Autodesk Inventor part; units mm, degrees
(part 2 of 3)
  line L885 (25.1106, 23.169) -> (25.1155, 23.1808)
  line L886 (25.1155, 23.1808) -> (25.12, 23.1924)
  line L887 (25.12, 23.1924) -> (25.124, 23.2037)
  line L888 (25.124, 23.2037) -> (25.1305, 23.2253)
  line L889 (25.1305, 23.2253) -> (25.1354, 23.2453)
  line L890 (25.1354, 23.2453) -> (25.1389, 23.2633)
  line L891 (25.1389, 23.2633) -> (25.1413, 23.2789)
  line L892 (25.1413, 23.2789) -> (25.1427, 23.2917)
  line L893 (25.1427, 23.2917) -> (25.1435, 23.3013)
  line L894 (25.1435, 23.3013) -> (25.1438, 23.3095)
  line L895 (25.1438, 23.3095) -> (25.1438, 23.4153)
  line L896 (25.1438, 23.4153) -> (25.1421, 23.4381)
  line L897 (25.1421, 23.4381) -> (25.138, 23.4642)
  line L898 (25.138, 23.4642) -> (25.1302, 23.498)
  line L899 (25.1302, 23.498) -> (25.1171, 23.5381)
  line L900 (25.1171, 23.5381) -> (25.0978, 23.5828)
  line L901 (25.0978, 23.5828) -> (25.0707, 23.6306)
  line L902 (25.0707, 23.6306) -> (25.0539, 23.6551)
  line L903 (25.0539, 23.6551) -> (25.0347, 23.6799)
  line L904 (25.0347, 23.6799) -> (25.0129, 23.7047)
  line L905 (25.0129, 23.7047) -> (24.9884, 23.7293)
  line L906 (24.9884, 23.7293) -> (24.961, 23.7535)
  line L907 (24.961, 23.7535) -> (24.9306, 23.7771)
  line L908 (24.9306, 23.7771) -> (24.897, 23.7999)
  line L909 (24.897, 23.7999) -> (24.8601, 23.8218)
  line L910 (24.8601, 23.8218) -> (24.8196, 23.8425)
  line L911 (24.8196, 23.8425) -> (24.7754, 23.8618)
  line L912 (24.7754, 23.8618) -> (24.7275, 23.8796)
  line L913 (24.7275, 23.8796) -> (24.6755, 23.8957)
  line L914 (24.6755, 23.8957) -> (24.6193, 23.9098)
  line L915 (24.6193, 23.9098) -> (24.5589, 23.9218)
  line L916 (24.5589, 23.9218) -> (24.4939, 23.9314)
  line L917 (24.4939, 23.9314) -> (24.4244, 23.9385)
  line L918 (24.4244, 23.9385) -> (24.35, 23.943)
  line L919 (24.35, 23.943) -> (24.2707, 23.9445)
  line L920 (24.2707, 23.9445) -> (21.0957, 23.9445)
  line L921 (21.0957, 23.9445) -> (21.0324, 23.9439)
  line L922 (21.0324, 23.9439) -> (20.9716, 23.9419)
  line L923 (20.9716, 23.9419) -> (20.9132, 23.9386)
  line L924 (20.9132, 23.9386) -> (20.8571, 23.9337)
  line L925 (20.8571, 23.9337) -> (20.8034, 23.9274)
  line L926 (20.8034, 23.9274) -> (20.752, 23.9194)
  line L927 (20.752, 23.9194) -> (20.7028, 23.9097)
  line L928 (20.7028, 23.9097) -> (20.6558, 23.8982)
  line L929 (20.6558, 23.8982) -> (20.611, 23.8848)
  line L930 (20.611, 23.8848) -> (20.5683, 23.8696)
  line L931 (20.5683, 23.8696) -> (20.5277, 23.8523)
  line L932 (20.5277, 23.8523) -> (20.4892, 23.8329)
  line L933 (20.4892, 23.8329) -> (20.4527, 23.8113)
  line L934 (20.4527, 23.8113) -> (20.4181, 23.7875)
  line L935 (20.4181, 23.7875) -> (20.3855, 23.7614)
  line L936 (20.3855, 23.7614) -> (20.3548, 23.7328)
  line L937 (20.3548, 23.7328) -> (20.3427, 23.7204)
  line L938 (20.3427, 23.7204) -> (20.3313, 23.7078)
  line L939 (20.3313, 23.7078) -> (20.3204, 23.6951)
  line L940 (20.3204, 23.6951) -> (20.31, 23.6823)
  line L941 (20.31, 23.6823) -> (20.3003, 23.6696)
  line L942 (20.3003, 23.6696) -> (20.2911, 23.6568)
  line L943 (20.2911, 23.6568) -> (20.2824, 23.6442)
  line L944 (20.2824, 23.6442) -> (20.2742, 23.6315)
  line L945 (20.2742, 23.6315) -> (20.2666, 23.619)
  line L946 (20.2666, 23.619) -> (20.2594, 23.6067)
  line L947 (20.2594, 23.6067) -> (20.2465, 23.5826)
  line L948 (20.2465, 23.5826) -> (20.2353, 23.5595)
  line L949 (20.2353, 23.5595) -> (20.2259, 23.5377)
  line L950 (20.2259, 23.5377) -> (20.2179, 23.5174)
  line L951 (20.2179, 23.5174) -> (20.2114, 23.499)
  line L952 (20.2114, 23.499) -> (20.2063, 23.4826)
  line L953 (20.2063, 23.4826) -> (20.2023, 23.4687)
  line L954 (20.2023, 23.4687) -> (20.1975, 23.4489)
  line L955 (20.1975, 23.4489) -> (20.1961, 23.4418)
  line L956 (20.1961, 23.4418) -> (20.1961, 22.8068)
  line L957 (19.7728, 22.8068) -> (19.7728, 23.4418)
  line L958 (19.7728, 23.4418) -> (19.7733, 23.4647)
  line L959 (19.7733, 23.4647) -> (19.7769, 23.5108)
  line L960 (19.7769, 23.5108) -> (19.7808, 23.5414)
  line L961 (19.7808, 23.5414) -> (19.7867, 23.5762)
  line L962 (19.7867, 23.5762) -> (19.7949, 23.6148)
  line L963 (19.7949, 23.6148) -> (19.8058, 23.6568)
  line L964 (19.8058, 23.6568) -> (19.8198, 23.7015)
  line L965 (19.8198, 23.7015) -> (19.8373, 23.7485)
  line L966 (19.8373, 23.7485) -> (19.8587, 23.7973)
  line L967 (19.8587, 23.7973) -> (19.8844, 23.8473)
  line L968 (19.8844, 23.8473) -> (19.9147, 23.8982)
  line L969 (19.9147, 23.8982) -> (19.95, 23.9493)
  line L970 (19.95, 23.9493) -> (19.9697, 23.9748)
  line L971 (19.9697, 23.9748) -> (19.9908, 24.0002)
  line L972 (19.9908, 24.0002) -> (20.0133, 24.0254)
  line L973 (20.0133, 24.0254) -> (20.0373, 24.0503)
  line L974 (20.0373, 24.0503) -> (20.0832, 24.0937)
  line L975 (20.0832, 24.0937) -> (20.1316, 24.1346)
  line L976 (20.1316, 24.1346) -> (20.1826, 24.1729)
  line L977 (20.1826, 24.1729) -> (20.2362, 24.2087)
  line L978 (20.2362, 24.2087) -> (20.2924, 24.2418)
  line L979 (20.2924, 24.2418) -> (20.3513, 24.2722)
  line L980 (20.3513, 24.2722) -> (20.4129, 24.2999)
  line L981 (20.4129, 24.2999) -> (20.4772, 24.3248)
  line L982 (20.4772, 24.3248) -> (20.5443, 24.347)
  line L983 (20.5443, 24.347) -> (20.6143, 24.3663)
  line L984 (20.6143, 24.3663) -> (20.6871, 24.3828)
  line L985 (20.6871, 24.3828) -> (20.7629, 24.3964)
  line L986 (20.7629, 24.3964) -> (20.8416, 24.407)
  line L987 (20.8416, 24.407) -> (20.9232, 24.4146)
  line L988 (20.9232, 24.4146) -> (21.0079, 24.4192)
  line L989 (21.0079, 24.4192) -> (21.0957, 24.4207)
  line L990 (21.0957, 24.4207) -> (24.2707, 24.4207)
  line L991 (24.2707, 24.4207) -> (24.3587, 24.4192)
  line L992 (28.4246, 20.8753) -> (27.9748, 20.8753)
  line L993 (27.9748, 20.8753) -> (27.9748, 23.6799)
  line L994 (27.9748, 23.6799) -> (26.7842, 22.3041)
  line L995 (26.7842, 22.3041) -> (26.2021, 22.3041)
  line L996 (26.2021, 22.3041) -> (28.0278, 24.3943)
  line L997 (28.0278, 24.3943) -> (28.4246, 24.3943)
  line L998 (28.4246, 24.3943) -> (28.4246, 20.8753)
  line L999 (36.3621, 21.4045) -> (40.86, 24.3149)
  line L1000 (40.86, 24.3149) -> (41.0982, 23.9445)
  line L1001 (41.0982, 23.9445) -> (38.9286, 22.5157)
  line L1002 (38.9286, 22.5157) -> (41.0982, 21.1135)
  line L1003 (41.0982, 21.1135) -> (40.86, 20.743)
  line L1004 (40.86, 20.743) -> (38.5317, 22.2512)
  line L1005 (38.5317, 22.2512) -> (35.9123, 20.5843)
  line L1006 (35.9123, 20.5843) -> (35.9123, 24.3943)
  line L1007 (35.9123, 24.3943) -> (36.3621, 24.3943)
  line L1008 (36.3621, 24.3943) -> (36.3621, 21.4045)
  line L1009 (42.2056, 21.9858) -> (42.2536, 21.9836)
  line L1010 (42.2536, 21.9836) -> (42.3006, 21.9799)
  line L1011 (42.3006, 21.9799) -> (42.3465, 21.9748)
  line L1012 (42.3465, 21.9748) -> (42.3915, 21.9684)
  line L1013 (42.3915, 21.9684) -> (42.4355, 21.9608)
  line L1014 (42.4355, 21.9608) -> (42.4786, 21.9519)
  line L1015 (42.4786, 21.9519) -> (42.5207, 21.9419)
  line L1016 (42.5207, 21.9419) -> (42.6024, 21.9188)
  line L1017 (42.6024, 21.9188) -> (42.6807, 21.8917)
  line L1018 (42.6807, 21.8917) -> (42.7558, 21.8612)
  line L1019 (42.7558, 21.8612) -> (42.8279, 21.8278)
  line L1020 (42.8279, 21.8278) -> (42.8972, 21.7919)
  line L1021 (42.8972, 21.7919) -> (42.9639, 21.754)
  line L1022 (42.9639, 21.754) -> (43.0283, 21.7146)
  line L1023 (43.0283, 21.7146) -> (43.0904, 21.674)
  line L1024 (43.0904, 21.674) -> (43.2088, 21.5916)
  line L1025 (43.2088, 21.5916) -> (43.3207, 21.5103)
  line L1026 (43.3207, 21.5103) -> (43.4077, 21.4435)
  line L1027 (43.4077, 21.4435) -> (43.491, 21.3826)
  line L1028 (43.491, 21.3826) -> (43.5316, 21.3546)
  line L1029 (43.5316, 21.3546) -> (43.5718, 21.3285)
  line L1030 (43.5718, 21.3285) -> (43.6117, 21.3043)
  line L1031 (43.6117, 21.3043) -> (43.6514, 21.2821)
  line L1032 (43.6514, 21.2821) -> (43.6911, 21.2621)
  line L1033 (43.6911, 21.2621) -> (43.731, 21.2444)
  line L1034 (43.731, 21.2444) -> (43.7712, 21.2292)
  line L1035 (43.7712, 21.2292) -> (43.8118, 21.2164)
  line L1036 (43.8118, 21.2164) -> (43.8531, 21.2063)
  line L1037 (43.8531, 21.2063) -> (43.8951, 21.1989)
  line L1038 (43.8951, 21.1989) -> (43.9381, 21.1944)
  line L1039 (43.9381, 21.1944) -> (43.9821, 21.1928)
  line L1040 (43.9821, 21.1928) -> (44.0262, 21.1944)
  line L1041 (44.0262, 21.1944) -> (44.0692, 21.1989)
  line L1042 (44.0692, 21.1989) -> (44.1112, 21.2063)
  line L1043 (44.1112, 21.2063) -> (44.1525, 21.2164)
  line L1044 (44.1525, 21.2164) -> (44.1931, 21.2292)
  line L1045 (44.1931, 21.2292) -> (44.2333, 21.2444)
  line L1046 (44.2333, 21.2444) -> (44.2731, 21.2621)
  line L1047 (44.2731, 21.2621) -> (44.3129, 21.2821)
  line L1048 (44.3129, 21.2821) -> (44.3526, 21.3043)
  line L1049 (44.3526, 21.3043) -> (44.3924, 21.3285)
  line L1050 (44.3924, 21.3285) -> (44.4326, 21.3546)
  line L1051 (44.4326, 21.3546) -> (44.4733, 21.3826)
  line L1052 (44.4733, 21.3826) -> (44.5566, 21.4435)
  line L1053 (44.5566, 21.4435) -> (44.6436, 21.5103)
  line L1054 (44.6436, 21.5103) -> (44.7554, 21.5916)
  line L1055 (44.7554, 21.5916) -> (44.873, 21.674)
  line L1056 (44.873, 21.674) -> (44.9344, 21.7146)
  line L1057 (44.9344, 21.7146) -> (44.9975, 21.754)
  line L1058 (44.9975, 21.754) -> (45.0626, 21.7919)
  line L1059 (45.0626, 21.7919) -> (45.1298, 21.8278)
  line L1060 (45.1298, 21.8278) -> (45.1991, 21.8612)
  line L1061 (45.1991, 21.8612) -> (45.2707, 21.8917)
  line L1062 (45.2707, 21.8917) -> (45.3447, 21.9188)
  line L1063 (45.3447, 21.9188) -> (45.4212, 21.9419)
  line L1064 (45.4212, 21.9419) -> (45.5004, 21.9608)
  line L1065 (45.5004, 21.9608) -> (45.5823, 21.9748)
  line L1066 (45.5823, 21.9748) -> (45.6671, 21.9836)
  line L1067 (45.6671, 21.9836) -> (45.7548, 21.9866)
  line L1068 (45.7548, 21.9866) -> (46.2575, 21.9866)
  line L1069 (46.2575, 21.9866) -> (46.2575, 21.5368)
  line L1070 (46.2575, 21.5368) -> (45.7548, 21.5368)
  line L1071 (45.7548, 21.5368) -> (45.7228, 21.5362)
  line L1072 (45.7228, 21.5362) -> (45.6913, 21.5344)
  line L1073 (45.6913, 21.5344) -> (45.6601, 21.5314)
  line L1074 (45.6601, 21.5314) -> (45.6294, 21.5273)
  line L1075 (45.6294, 21.5273) -> (45.5991, 21.5222)
  line L1076 (45.5991, 21.5222) -> (45.5692, 21.516)
  line L1077 (45.5692, 21.516) -> (45.5105, 21.5008)
  line L1078 (45.5105, 21.5008) -> (45.4532, 21.482)
  line L1079 (45.4532, 21.482) -> (45.3972, 21.46)
  line L1080 (45.3972, 21.46) -> (45.3423, 21.4352)
  line L1081 (45.3423, 21.4352) -> (45.2885, 21.4078)
  line L1082 (45.2885, 21.4078) -> (45.2356, 21.3782)
  line L1083 (45.2356, 21.3782) -> (45.1836, 21.3469)
  line L1084 (45.1836, 21.3469) -> (45.1322, 21.314)
  line L1085 (45.1322, 21.314) -> (45.0814, 21.2801)
  line L1086 (45.0814, 21.2801) -> (44.8817, 21.1399)
  line L1087 (44.8817, 21.1399) -> (44.7822, 21.0621)
  line L1088 (44.7822, 21.0621) -> (44.732, 21.0247)
  line L1089 (44.732, 21.0247) -> (44.6812, 20.9886)
  line L1090 (44.6812, 20.9886) -> (44.6296, 20.9541)
  line L1091 (44.6296, 20.9541) -> (44.5771, 20.9213)
  line L1092 (44.5771, 20.9213) -> (44.5234, 20.8906)
  line L1093 (44.5234, 20.8906) -> (44.4683, 20.8621)
  line L1094 (44.4683, 20.8621) -> (44.4117, 20.8361)
  line L1095 (44.4117, 20.8361) -> (44.3533, 20.8128)
  line L1096 (44.3533, 20.8128) -> (44.293, 20.7924)
  line L1097 (44.293, 20.7924) -> (44.2306, 20.7753)
  line L1098 (44.2306, 20.7753) -> (44.1658, 20.7615)
  line L1099 (44.1658, 20.7615) -> (44.0986, 20.7514)
  line L1100 (44.0986, 20.7514) -> (44.0286, 20.7452)
  line L1101 (44.0286, 20.7452) -> (43.9557, 20.743)
  line L1102 (43.9557, 20.743) -> (43.9188, 20.7436)
  line L1103 (43.9188, 20.7436) -> (43.8828, 20.7455)
  line L1104 (43.8828, 20.7455) -> (43.8474, 20.7484)
  line L1105 (43.8474, 20.7484) -> (43.8128, 20.7525)
  line L1106 (43.8128, 20.7525) -> (43.7788, 20.7576)
  line L1107 (43.7788, 20.7576) -> (43.7455, 20.7638)
  line L1108 (43.7455, 20.7638) -> (43.6808, 20.779)
  line L1109 (43.6808, 20.779) -> (43.6183, 20.7978)
  line L1110 (43.6183, 20.7978) -> (43.558, 20.8198)
  line L1111 (43.558, 20.8198) -> (43.4997, 20.8446)
  line L1112 (43.4997, 20.8446) -> (43.443, 20.872)
  line L1113 (43.443, 20.872) -> (43.388, 20.9016)
  line L1114 (43.388, 20.9016) -> (43.3343, 20.9329)
  line L1115 (43.3343, 20.9329) -> (43.2817, 20.9658)
  line L1116 (43.2817, 20.9658) -> (43.2301, 20.9998)
  line L1117 (43.2301, 20.9998) -> (43.1291, 21.0697)
  line L1118 (43.1291, 21.0697) -> (43.0296, 21.1399)
  line L1119 (43.0296, 21.1399) -> (42.9313, 21.2177)
  line L1120 (42.9313, 21.2177) -> (42.8337, 21.2912)
  line L1121 (42.8337, 21.2912) -> (42.7845, 21.3257)
  line L1122 (42.7845, 21.3257) -> (42.7348, 21.3585)
  line L1123 (42.7348, 21.3585) -> (42.6843, 21.3892)
  line L1124 (42.6843, 21.3892) -> (42.6328, 21.4177)
  line L1125 (42.6328, 21.4177) -> (42.58, 21.4437)
  line L1126 (42.58, 21.4437) -> (42.5258, 21.467)
  line L1127 (42.5258, 21.467) -> (42.4699, 21.4874)
  line L1128 (42.4699, 21.4874) -> (42.412, 21.5045)
  line L1129 (42.412, 21.5045) -> (42.352, 21.5183)
  line L1130 (42.352, 21.5183) -> (42.2895, 21.5284)
  line L1131 (42.2895, 21.5284) -> (42.2244, 21.5347)
  line L1132 (42.2244, 21.5347) -> (42.1565, 21.5368)
  line L1133 (42.1565, 21.5368) -> (41.6538, 21.5368)
  line L1134 (41.6538, 21.5368) -> (41.6538, 21.9866)
  line L1135 (41.6538, 21.9866) -> (42.1565, 21.9866)
  line L1136 (42.1565, 21.9866) -> (42.2056, 21.9858)
  line L1137 (35.2244, 23.9974) -> (29.9592, 23.9974)
  line L1138 (29.9592, 23.9974) -> (29.9942, 23.8886)
  line L1139 (29.9942, 23.8886) -> (30.0411, 23.7622)
  line L1140 (30.0411, 23.7622) -> (30.1015, 23.6202)
  line L1141 (30.1015, 23.6202) -> (30.1375, 23.5441)
  line L1142 (30.1375, 23.5441) -> (30.1775, 23.4649)
  line L1143 (30.1775, 23.4649) -> (30.2219, 23.383)
  line L1144 (30.2219, 23.383) -> (30.2708, 23.2985)
  line L1145 (30.2708, 23.2985) -> (30.3246, 23.2118)
  line L1146 (30.3246, 23.2118) -> (30.3834, 23.123)
  line L1147 (30.3834, 23.123) -> (30.4474, 23.0326)
  line L1148 (30.4474, 23.0326) -> (30.517, 22.9408)
  line L1149 (30.517, 22.9408) -> (30.5923, 22.8478)
  line L1150 (30.5923, 22.8478) -> (30.6736, 22.7539)
  line L1151 (30.6736, 22.7539) -> (30.7495, 22.6708)
  line L1152 (30.7495, 22.6708) -> (30.8286, 22.5902)
  line L1153 (30.8286, 22.5902) -> (30.9106, 22.512)
  line L1154 (30.9106, 22.512) -> (30.9956, 22.4364)
  line L1155 (30.9956, 22.4364) -> (31.0836, 22.3632)
  line L1156 (31.0836, 22.3632) -> (31.1745, 22.2925)
  line L1157 (31.1745, 22.2925) -> (31.2682, 22.2243)
  line L1158 (31.2682, 22.2243) -> (31.3648, 22.1586)
  line L1159 (31.3648, 22.1586) -> (31.4642, 22.0953)
  line L1160 (31.4642, 22.0953) -> (31.5663, 22.0345)
  line L1161 (31.5663, 22.0345) -> (31.6711, 21.9762)
  line L1162 (31.6711, 21.9762) -> (31.7786, 21.9204)
  line L1163 (31.7786, 21.9204) -> (31.8888, 21.8671)
  line L1164 (31.8888, 21.8671) -> (32.0015, 21.8163)
  line L1165 (32.0015, 21.8163) -> (32.1168, 21.7679)
  line L1166 (32.1168, 21.7679) -> (32.2346, 21.722)
  line L1167 (32.2346, 21.722) -> (32.5485, 21.6092)
  line L1168 (32.5485, 21.6092) -> (32.8754, 21.5095)
  line L1169 (32.8754, 21.5095) -> (33.0439, 21.4647)
  line L1170 (33.0439, 21.4647) -> (33.216, 21.4234)
  line L1171 (33.216, 21.4234) -> (33.3915, 21.3857)
  line L1172 (33.3915, 21.3857) -> (33.5708, 21.3516)
  line L1173 (33.5708, 21.3516) -> (33.7537, 21.3212)
  line L1174 (33.7537, 21.3212) -> (33.9405, 21.2946)
  line L1175 (33.9405, 21.2946) -> (34.1311, 21.2719)
  line L1176 (34.1311, 21.2719) -> (34.3257, 21.2532)
  line L1177 (34.3257, 21.2532) -> (34.5243, 21.2385)
  line L1178 (34.5243, 21.2385) -> (34.727, 21.2279)
  line L1179 (34.727, 21.2279) -> (34.9339, 21.2214)
  line L1180 (34.9339, 21.2214) -> (35.145, 21.2193)
  line L1181 (35.145, 21.2193) -> (35.2509, 21.2193)
  line L1182 (35.2509, 21.2193) -> (35.2509, 20.7695)
  line L1183 (35.2509, 20.7695) -> (35.145, 20.7695)
  line L1184 (35.145, 20.7695) -> (34.9283, 20.7717)
  line L1185 (34.9283, 20.7717) -> (34.7147, 20.7781)
  line L1186 (34.7147, 20.7781) -> (34.5043, 20.7889)
  line L1187 (34.5043, 20.7889) -> (34.2971, 20.8038)
  line L1188 (34.2971, 20.8038) -> (34.0932, 20.8229)
  line L1189 (34.0932, 20.8229) -> (33.8926, 20.8462)
  line L1190 (33.8926, 20.8462) -> (33.6953, 20.8736)
  line L1191 (33.6953, 20.8736) -> (33.5013, 20.9051)
  line L1192 (33.5013, 20.9051) -> (33.3108, 20.9406)
  line L1193 (33.3108, 20.9406) -> (33.1237, 20.9801)
  line L1194 (33.1237, 20.9801) -> (32.9401, 21.0235)
  line L1195 (32.9401, 21.0235) -> (32.7601, 21.0709)
  line L1196 (32.7601, 21.0709) -> (32.5836, 21.1221)
  line L1197 (32.5836, 21.1221) -> (32.4107, 21.1772)
  line L1198 (32.4107, 21.1772) -> (32.2414, 21.236)
  line L1199 (32.2414, 21.236) -> (32.0759, 21.2987)
  line L1200 (32.0759, 21.2987) -> (31.9438, 21.3542)
  line L1201 (31.9438, 21.3542) -> (31.8153, 21.4116)
  line L1202 (31.8153, 21.4116) -> (31.6904, 21.4711)
  line L1203 (31.6904, 21.4711) -> (31.569, 21.5327)
  line L1204 (31.569, 21.5327) -> (31.451, 21.5964)
  line L1205 (31.451, 21.5964) -> (31.3364, 21.6624)
  line L1206 (31.3364, 21.6624) -> (31.225, 21.7307)
  line L1207 (31.225, 21.7307) -> (31.1168, 21.8014)
  line L1208 (31.1168, 21.8014) -> (31.0116, 21.8746)
  line L1209 (31.0116, 21.8746) -> (30.9095, 21.9503)
  line L1210 (30.9095, 21.9503) -> (30.8104, 22.0287)
  line L1211 (30.8104, 22.0287) -> (30.7141, 22.1098)
  line L1212 (30.7141, 22.1098) -> (30.6206, 22.1937)
  line L1213 (30.6206, 22.1937) -> (30.5298, 22.2804)
  line L1214 (30.5298, 22.2804) -> (30.4417, 22.3701)
  line L1215 (30.4417, 22.3701) -> (30.3561, 22.4628)
  line L1216 (30.3561, 22.4628) -> (30.2861, 22.5422)
  line L1217 (30.2861, 22.5422) -> (30.2198, 22.6214)
  line L1218 (30.2198, 22.6214) -> (30.1573, 22.7003)
  line L1219 (30.1573, 22.7003) -> (30.0983, 22.7787)
  line L1220 (30.0983, 22.7787) -> (30.0427, 22.8566)
  line L1221 (30.0427, 22.8566) -> (29.9906, 22.9337)
  line L1222 (29.9906, 22.9337) -> (29.9417, 23.0099)
  line L1223 (29.9417, 23.0099) -> (29.896, 23.085)
  line L1224 (29.896, 23.085) -> (29.8533, 23.159)
  line L1225 (29.8533, 23.159) -> (29.8136, 23.2315)
  line L1226 (29.8136, 23.2315) -> (29.7426, 23.3721)
  line L1227 (29.7426, 23.3721) -> (29.6823, 23.5054)
  line L1228 (29.6823, 23.5054) -> (29.6318, 23.6303)
  line L1229 (29.6318, 23.6303) -> (29.5903, 23.7456)
  line L1230 (29.5903, 23.7456) -> (29.5569, 23.8501)
  line L1231 (29.5569, 23.8501) -> (29.5309, 23.9425)
  line L1232 (29.5309, 23.9425) -> (29.5115, 24.0218)
  line L1233 (29.5115, 24.0218) -> (29.4978, 24.0866)
  line L1234 (29.4978, 24.0866) -> (29.489, 24.1359)
  line L1235 (29.489, 24.1359) -> (29.483, 24.1826)
  line L1236 (29.483, 24.1826) -> (29.4565, 24.3943)
  line L1237 (29.4565, 24.3943) -> (35.2244, 24.3943)
  line L1238 (35.2244, 24.3943) -> (35.2244, 23.9974)
  line L1239 (12.6069, 24.3657) -> (12.6892, 24.3591)
  line L1240 (12.6892, 24.3591) -> (12.7701, 24.3483)
  line L1241 (12.7701, 24.3483) -> (12.8493, 24.3331)
  line L1242 (12.8493, 24.3331) -> (12.9269, 24.3136)
  line L1243 (12.9269, 24.3136) -> (13.0027, 24.2897)
  line L1244 (13.0027, 24.2897) -> (13.0765, 24.2615)
  line L1245 (13.0765, 24.2615) -> (13.1482, 24.2289)
  line L1246 (13.1482, 24.2289) -> (13.2178, 24.192)
  line L1247 (13.2178, 24.192) -> (13.2851, 24.1508)
  line L1248 (13.2851, 24.1508) -> (13.35, 24.1052)
  line L1249 (13.35, 24.1052) -> (13.4124, 24.0553)
  line L1250 (13.4124, 24.0553) -> (13.4722, 24.001)
  line L1251 (13.4722, 24.001) -> (13.5292, 23.9424)
  line L1252 (13.5292, 23.9424) -> (13.5833, 23.8795)
  line L1253 (13.5833, 23.8795) -> (13.6344, 23.8122)
  line L1254 (13.6344, 23.8122) -> (13.6682, 23.7626)
  line L1255 (13.6682, 23.7626) -> (13.7001, 23.7134)
  line L1256 (13.7001, 23.7134) -> (13.7301, 23.6649)
  line L1257 (13.7301, 23.6649) -> (13.758, 23.6175)
  line L1258 (13.758, 23.6175) -> (13.784, 23.5714)
  line L1259 (13.784, 23.5714) -> (13.8079, 23.5271)
  line L1260 (13.8079, 23.5271) -> (13.8297, 23.4849)
  line L1261 (13.8297, 23.4849) -> (13.8494, 23.4451)
  line L1262 (13.8494, 23.4451) -> (13.8669, 23.4081)
  line L1263 (13.8669, 23.4081) -> (13.8822, 23.3742)
  line L1264 (13.8822, 23.3742) -> (13.8953, 23.3439)
  line L1265 (13.8953, 23.3439) -> (13.906, 23.3173)
  line L1266 (13.906, 23.3173) -> (13.9145, 23.295)
  line L1267 (13.9145, 23.295) -> (13.9206, 23.2772)
  line L1268 (13.9206, 23.2772) -> (13.9242, 23.2643)
  line L1269 (13.9242, 23.2643) -> (13.9255, 23.2566)
  line L1270 (13.9255, 23.2566) -> (13.9255, 23.1772)
  line L1271 (13.9255, 23.1772) -> (13.5021, 23.0449)
  line L1272 (13.5021, 23.0449) -> (13.4757, 23.1507)
  line L1273 (13.4757, 23.1507) -> (13.4649, 23.1908)
  line L1274 (13.4649, 23.1908) -> (13.4506, 23.2359)
  line L1275 (13.4506, 23.2359) -> (13.4294, 23.293)
  line L1276 (13.4294, 23.293) -> (13.416, 23.325)
  line L1277 (13.416, 23.325) -> (13.4007, 23.3587)
  line L1278 (13.4007, 23.3587) -> (13.3834, 23.3938)
  line L1279 (13.3834, 23.3938) -> (13.364, 23.4298)
  line L1280 (13.364, 23.4298) -> (13.3425, 23.4662)
  line L1281 (13.3425, 23.4662) -> (13.3187, 23.5027)
  line L1282 (13.3187, 23.5027) -> (13.2925, 23.5388)
  line L1283 (13.2925, 23.5388) -> (13.264, 23.5741)
  line L1284 (13.264, 23.5741) -> (13.224, 23.6221)
  line L1285 (13.224, 23.6221) -> (13.1833, 23.6671)
  line L1286 (13.1833, 23.6671) -> (13.142, 23.709)
  line L1287 (13.142, 23.709) -> (13.0999, 23.7477)
  line L1288 (13.0999, 23.7477) -> (13.057, 23.7834)
  line L1289 (13.057, 23.7834) -> (13.0133, 23.8159)
  line L1290 (13.0133, 23.8159) -> (12.9688, 23.8454)
  line L1291 (12.9688, 23.8454) -> (12.9234, 23.8717)
  line L1292 (12.9234, 23.8717) -> (12.877, 23.895)
  line L1293 (12.877, 23.895) -> (12.8297, 23.9151)
  line L1294 (12.8297, 23.9151) -> (12.7813, 23.9322)
  line L1295 (12.7813, 23.9322) -> (12.7319, 23.9461)
  line L1296 (12.7319, 23.9461) -> (12.6815, 23.957)
  line L1297 (12.6815, 23.957) -> (12.6299, 23.9647)
  line L1298 (12.6299, 23.9647) -> (12.5771, 23.9694)
  line L1299 (12.5771, 23.9694) -> (12.5232, 23.971)
  line L1300 (12.5232, 23.971) -> (9.3746, 23.971)
  line L1301 (9.3746, 23.971) -> (9.2976, 23.9695)
  line L1302 (9.2976, 23.9695) -> (9.2253, 23.9653)
  line L1303 (9.2253, 23.9653) -> (9.1575, 23.9585)
  line L1304 (9.1575, 23.9585) -> (9.094, 23.9493)
  line L1305 (9.094, 23.9493) -> (9.0348, 23.9379)
  line L1306 (9.0348, 23.9379) -> (8.9797, 23.9244)
  line L1307 (8.9797, 23.9244) -> (8.9284, 23.909)
  line L1308 (8.9284, 23.909) -> (8.881, 23.892)
  line L1309 (8.881, 23.892) -> (8.8372, 23.8734)
  line L1310 (8.8372, 23.8734) -> (8.7969, 23.8535)
  line L1311 (8.7969, 23.8535) -> (8.76, 23.8325)
  line L1312 (8.76, 23.8325) -> (8.7263, 23.8105)
  line L1313 (8.7263, 23.8105) -> (8.6956, 23.7877)
  line L1314 (8.6956, 23.7877) -> (8.6679, 23.7643)
  line L1315 (8.6679, 23.7643) -> (8.6429, 23.7404)
  line L1316 (8.6429, 23.7404) -> (8.6206, 23.7163)
  line L1317 (8.6206, 23.7163) -> (8.6007, 23.6921)
  line L1318 (8.6007, 23.6921) -> (8.5832, 23.668)
  line L1319 (8.5832, 23.668) -> (8.5678, 23.6442)
  line L1320 (8.5678, 23.6442) -> (8.5545, 23.6208)
  line L1321 (8.5545, 23.6208) -> (8.5431, 23.5981)
  line L1322 (8.5431, 23.5981) -> (8.5335, 23.5762)
  line L1323 (8.5335, 23.5762) -> (8.5189, 23.5356)
  line L1324 (8.5189, 23.5356) -> (8.5095, 23.5004)
  line L1325 (8.5095, 23.5004) -> (8.5043, 23.4721)
  line L1326 (8.5043, 23.4721) -> (8.5015, 23.4418)
  line L1327 (8.5015, 23.4418) -> (8.5015, 23.336)
  line L1328 (8.5015, 23.336) -> (8.5032, 23.3132)
  line L1329 (8.5032, 23.3132) -> (8.5073, 23.2871)
  line L1330 (8.5073, 23.2871) -> (8.5151, 23.2533)
  line L1331 (8.5151, 23.2533) -> (8.5281, 23.2132)
  line L1332 (8.5281, 23.2132) -> (8.5475, 23.1685)
  line L1333 (8.5475, 23.1685) -> (8.5746, 23.1207)
  line L1334 (8.5746, 23.1207) -> (8.5914, 23.0961)
  line L1335 (8.5914, 23.0961) -> (8.6106, 23.0714)
  line L1336 (8.6106, 23.0714) -> (8.6324, 23.0466)
  line L1337 (8.6324, 23.0466) -> (8.6569, 23.022)
  line L1338 (8.6569, 23.022) -> (8.6843, 22.9978)
  line L1339 (8.6843, 22.9978) -> (8.7147, 22.9742)
  line L1340 (8.7147, 22.9742) -> (8.7483, 22.9514)
  line L1341 (8.7483, 22.9514) -> (8.7852, 22.9295)
  line L1342 (8.7852, 22.9295) -> (8.8257, 22.9088)
  line L1343 (8.8257, 22.9088) -> (8.8699, 22.8895)
  line L1344 (8.8699, 22.8895) -> (8.9178, 22.8717)
  line L1345 (8.9178, 22.8717) -> (8.9698, 22.8556)
  line L1346 (8.9698, 22.8556) -> (9.026, 22.8415)
  line L1347 (9.026, 22.8415) -> (9.0864, 22.8295)
  line L1348 (9.0864, 22.8295) -> (9.1514, 22.8199)
  line L1349 (9.1514, 22.8199) -> (9.2209, 22.8127)
  line L1350 (9.2209, 22.8127) -> (9.2953, 22.8083)
  line L1351 (9.2953, 22.8083) -> (9.3746, 22.8068)
  line L1352 (9.3746, 22.8068) -> (12.5761, 22.8068)
  line L1353 (12.5761, 22.8068) -> (12.6641, 22.8052)
  line L1354 (12.6641, 22.8052) -> (12.7496, 22.8006)
  line L1355 (12.7496, 22.8006) -> (12.8325, 22.793)
  line L1356 (12.8325, 22.793) -> (12.9126, 22.7824)
  line L1357 (12.9126, 22.7824) -> (12.9899, 22.7688)
  line L1358 (12.9899, 22.7688) -> (13.0644, 22.7524)
  line L1359 (13.0644, 22.7524) -> (13.136, 22.733)
  line L1360 (13.136, 22.733) -> (13.2045, 22.7109)
  line L1361 (13.2045, 22.7109) -> (13.2699, 22.6859)
  line L1362 (13.2699, 22.6859) -> (13.3321, 22.6582)
  line L1363 (13.3321, 22.6582) -> (13.3911, 22.6278)
  line L1364 (13.3911, 22.6278) -> (13.4467, 22.5947)
  line L1365 (13.4467, 22.5947) -> (13.499, 22.559)
  line L1366 (13.499, 22.559) -> (13.5477, 22.5207)
  line L1367 (13.5477, 22.5207) -> (13.5929, 22.4798)
  line L1368 (13.5929, 22.4798) -> (13.6344, 22.4364)
  line L1369 (13.6344, 22.4364) -> (13.6585, 22.4114)
  line L1370 (13.6585, 22.4114) -> (13.681, 22.3862)
  line L1371 (13.681, 22.3862) -> (13.7021, 22.3608)
  line L1372 (13.7021, 22.3608) -> (13.7218, 22.3353)
  line L1373 (13.7218, 22.3353) -> (13.7401, 22.3098)
  line L1374 (13.7401, 22.3098) -> (13.7571, 22.2842)
  line L1375 (13.7571, 22.2842) -> (13.7728, 22.2587)
  line L1376 (13.7728, 22.2587) -> (13.7874, 22.2334)
  line L1377 (13.7874, 22.2334) -> (13.8008, 22.2082)
  line L1378 (13.8008, 22.2082) -> (13.813, 22.1833)
  line L1379 (13.813, 22.1833) -> (13.8242, 22.1587)
  line L1380 (13.8242, 22.1587) -> (13.8344, 22.1345)
  line L1381 (13.8344, 22.1345) -> (13.8519, 22.0875)
  line L1382 (13.8519, 22.0875) -> (13.8659, 22.0428)
  line L1383 (13.8659, 22.0428) -> (13.8768, 22.0009)
  line L1384 (13.8768, 22.0009) -> (13.885, 21.9622)
  line L1385 (13.885, 21.9622) -> (13.8909, 21.9274)
  line L1386 (13.8909, 21.9274) -> (13.8949, 21.8969)
  line L1387 (13.8949, 21.8969) -> (13.8973, 21.8711)
  line L1388 (13.8973, 21.8711) -> (13.8985, 21.8507)
  line L1389 (13.8985, 21.8507) -> (13.899, 21.8278)
  line L1390 (13.899, 21.8278) -> (13.899, 21.722)
  line L1391 (13.899, 21.722) -> (13.8985, 21.6991)
  line L1392 (13.8985, 21.6991) -> (13.8949, 21.653)
  line L1393 (13.8949, 21.653) -> (13.8909, 21.6224)
  line L1394 (13.8909, 21.6224) -> (13.885, 21.5876)
  line L1395 (13.885, 21.5876) -> (13.8768, 21.5489)
  line L1396 (13.8768, 21.5489) -> (13.8659, 21.507)
  line L1397 (13.8659, 21.507) -> (13.8519, 21.4623)
  line L1398 (13.8519, 21.4623) -> (13.8344, 21.4153)
  line L1399 (13.8344, 21.4153) -> (13.813, 21.3665)
  line L1400 (13.813, 21.3665) -> (13.7874, 21.3164)
  line L1401 (13.7874, 21.3164) -> (13.7571, 21.2656)
  line L1402 (13.7571, 21.2656) -> (13.7218, 21.2145)
  line L1403 (13.7218, 21.2145) -> (13.7021, 21.189)
  line L1404 (13.7021, 21.189) -> (13.681, 21.1636)
  line L1405 (13.681, 21.1636) -> (13.6585, 21.1384)
  line L1406 (13.6585, 21.1384) -> (13.6344, 21.1134)
  line L1407 (13.6344, 21.1134) -> (13.5885, 21.0747)
  line L1408 (13.5885, 21.0747) -> (13.5401, 21.0379)
  line L1409 (13.5401, 21.0379) -> (13.4891, 21.0031)
  line L1410 (13.4891, 21.0031) -> (13.4356, 20.9704)
  line L1411 (13.4356, 20.9704) -> (13.3794, 20.9399)
  line L1412 (13.3794, 20.9399) -> (13.3205, 20.9116)
  line L1413 (13.3205, 20.9116) -> (13.2589, 20.8856)
  line L1414 (13.2589, 20.8856) -> (13.1945, 20.8621)
  line L1415 (13.1945, 20.8621) -> (13.1274, 20.841)
  line L1416 (13.1274, 20.841) -> (13.0575, 20.8225)
  line L1417 (13.0575, 20.8225) -> (12.9846, 20.8066)
  line L1418 (12.9846, 20.8066) -> (12.9089, 20.7935)
  line L1419 (12.9089, 20.7935) -> (12.8302, 20.7831)
  line L1420 (12.8302, 20.7831) -> (12.7485, 20.7756)
  line L1421 (12.7485, 20.7756) -> (12.6638, 20.771)
  line L1422 (12.6638, 20.771) -> (12.5761, 20.7695)
  line L1423 (12.5761, 20.7695) -> (9.4805, 20.7695)
  line L1424 (9.4805, 20.7695) -> (9.3968, 20.7717)
  line L1425 (9.3968, 20.7717) -> (9.3144, 20.7782)
  line L1426 (9.3144, 20.7782) -> (9.2336, 20.789)
  line L1427 (9.2336, 20.789) -> (9.1543, 20.8042)
  line L1428 (9.1543, 20.8042) -> (9.0767, 20.8238)
  line L1429 (9.0767, 20.8238) -> (9.001, 20.8476)
  line L1430 (9.001, 20.8476) -> (8.9271, 20.8758)
  line L1431 (8.9271, 20.8758) -> (8.8554, 20.9084)
  line L1432 (8.8554, 20.9084) -> (8.7858, 20.9453)
  line L1433 (8.7858, 20.9453) -> (8.7185, 20.9865)
  line L1434 (8.7185, 20.9865) -> (8.6536, 21.0321)
  line L1435 (8.6536, 21.0321) -> (8.5912, 21.082)
  line L1436 (8.5912, 21.082) -> (8.5315, 21.1363)
  line L1437 (8.5315, 21.1363) -> (8.4745, 21.1949)
  line L1438 (8.4745, 21.1949) -> (8.4204, 21.2578)
  line L1439 (8.4204, 21.2578) -> (8.3692, 21.3251)
  line L1440 (8.3692, 21.3251) -> (8.3354, 21.3747)
  line L1441 (8.3354, 21.3747) -> (8.3035, 21.4239)
  line L1442 (8.3035, 21.4239) -> (8.2736, 21.4724)
  line L1443 (8.2736, 21.4724) -> (8.2456, 21.5198)
  line L1444 (8.2456, 21.5198) -> (8.2196, 21.5659)
  line L1445 (8.2196, 21.5659) -> (8.1957, 21.6102)
  line L1446 (8.1957, 21.6102) -> (8.1739, 21.6524)
  line L1447 (8.1739, 21.6524) -> (8.1542, 21.6922)
  line L1448 (8.1542, 21.6922) -> (8.1367, 21.7292)
  line L1449 (8.1367, 21.7292) -> (8.1214, 21.7631)
  line L1450 (8.1214, 21.7631) -> (8.1084, 21.7934)
  line L1451 (8.1084, 21.7934) -> (8.0976, 21.82)
  line L1452 (8.0976, 21.82) -> (8.0892, 21.8423)
  line L1453 (8.0892, 21.8423) -> (8.0831, 21.8601)
  line L1454 (8.0831, 21.8601) -> (8.0794, 21.873)
  line L1455 (8.0794, 21.873) -> (8.0782, 21.8807)
  line L1456 (8.0782, 21.8807) -> (8.0517, 21.9866)
  line L1457 (8.0517, 21.9866) -> (8.5015, 22.0924)
  line L1458 (8.5015, 22.0924) -> (8.528, 21.9866)
  line L1459 (8.528, 21.9866) -> (8.5387, 21.9465)
  line L1460 (8.5387, 21.9465) -> (8.5531, 21.9015)
  line L1461 (8.5531, 21.9015) -> (8.5743, 21.8444)
  line L1462 (8.5743, 21.8444) -> (8.5876, 21.8123)
  line L1463 (8.5876, 21.8123) -> (8.6029, 21.7786)
  line L1464 (8.6029, 21.7786) -> (8.6202, 21.7435)
  line L1465 (8.6202, 21.7435) -> (8.6396, 21.7075)
  line L1466 (8.6396, 21.7075) -> (8.6611, 21.6711)
  line L1467 (8.6611, 21.6711) -> (8.685, 21.6346)
  line L1468 (8.685, 21.6346) -> (8.7111, 21.5985)
  line L1469 (8.7111, 21.5985) -> (8.7396, 21.5632)
  line L1470 (8.7396, 21.5632) -> (8.7796, 21.5152)
  line L1471 (8.7796, 21.5152) -> (8.8203, 21.4702)
  line L1472 (8.8203, 21.4702) -> (8.8617, 21.4284)
  line L1473 (8.8617, 21.4284) -> (8.9038, 21.3896)
  line L1474 (8.9038, 21.3896) -> (8.9466, 21.354)
  line L1475 (8.9466, 21.354) -> (8.9903, 21.3214)
  line L1476 (8.9903, 21.3214) -> (9.0348, 21.2919)
  line L1477 (9.0348, 21.2919) -> (9.0803, 21.2656)
  line L1478 (9.0803, 21.2656) -> (9.1266, 21.2423)
  line L1479 (9.1266, 21.2423) -> (9.174, 21.2222)
  line L1480 (9.174, 21.2222) -> (9.2223, 21.2051)
  line L1481 (9.2223, 21.2051) -> (9.2717, 21.1912)
  line L1482 (9.2717, 21.1912) -> (9.3222, 21.1803)
  line L1483 (9.3222, 21.1803) -> (9.3737, 21.1726)
  line L1484 (9.3737, 21.1726) -> (9.4265, 21.1679)
  line L1485 (9.4265, 21.1679) -> (9.4805, 21.1664)
  line L1486 (9.4805, 21.1664) -> (12.5232, 21.1664)
  line L1487 (12.5232, 21.1664) -> (12.5864, 21.167)
  line L1488 (12.5864, 21.167) -> (12.6472, 21.169)
  line L1489 (12.6472, 21.169) -> (12.7057, 21.1723)
  line L1490 (12.7057, 21.1723) -> (12.7617, 21.1771)
  line L1491 (12.7617, 21.1771) -> (12.8154, 21.1835)
  line L1492 (12.8154, 21.1835) -> (12.8669, 21.1915)
  line L1493 (12.8669, 21.1915) -> (12.9161, 21.2012)
  line L1494 (12.9161, 21.2012) -> (12.963, 21.2127)
  line L1495 (12.963, 21.2127) -> (13.0078, 21.226)
  line L1496 (13.0078, 21.226) -> (13.0505, 21.2413)
  line L1497 (13.0505, 21.2413) -> (13.0911, 21.2586)
  line L1498 (13.0911, 21.2586) -> (13.1296, 21.278)
  line L1499 (13.1296, 21.278) -> (13.1662, 21.2996)
  line L1500 (13.1662, 21.2996) -> (13.2007, 21.3234)
  line L1501 (13.2007, 21.3234) -> (13.2333, 21.3495)
  line L1502 (13.2333, 21.3495) -> (13.264, 21.378)
  line L1503 (13.264, 21.378) -> (13.2784, 21.3882)
  line L1504 (13.2784, 21.3882) -> (13.2919, 21.3987)
  line L1505 (13.2919, 21.3987) -> (13.3046, 21.4097)
  line L1506 (13.3046, 21.4097) -> (13.3164, 21.4209)
  line L1507 (13.3164, 21.4209) -> (13.3274, 21.4324)
  line L1508 (13.3274, 21.4324) -> (13.3376, 21.4442)
  line L1509 (13.3376, 21.4442) -> (13.3471, 21.4561)
  line L1510 (13.3471, 21.4561) -> (13.3558, 21.4682)
  line L1511 (13.3558, 21.4682) -> (13.3638, 21.4803)
  line L1512 (13.3638, 21.4803) -> (13.3712, 21.4924)
  line L1513 (13.3712, 21.4924) -> (13.3779, 21.5046)
  line L1514 (13.3779, 21.5046) -> (13.384, 21.5166)
  line L1515 (13.384, 21.5166) -> (13.3895, 21.5286)
  line L1516 (13.3895, 21.5286) -> (13.3945, 21.5404)
  line L1517 (13.3945, 21.5404) -> (13.3989, 21.5519)
  line L1518 (13.3989, 21.5519) -> (13.4029, 21.5632)
  line L1519 (13.4029, 21.5632) -> (13.4095, 21.5849)
  line L1520 (13.4095, 21.5849) -> (13.4144, 21.6049)
  line L1521 (13.4144, 21.6049) -> (13.4179, 21.6229)
  line L1522 (13.4179, 21.6229) -> (13.4203, 21.6385)
  line L1523 (13.4203, 21.6385) -> (13.4217, 21.6513)
  line L1524 (13.4217, 21.6513) -> (13.4224, 21.6609)
  line L1525 (13.4224, 21.6609) -> (13.4228, 21.6691)
  line L1526 (13.4228, 21.6691) -> (13.4228, 21.7749)
  line L1527 (13.4228, 21.7749) -> (13.421, 21.7976)
  line L1528 (13.421, 21.7976) -> (13.417, 21.8237)
  line L1529 (13.417, 21.8237) -> (13.4091, 21.8576)
  line L1530 (13.4091, 21.8576) -> (13.3961, 21.8976)
  line L1531 (13.3961, 21.8976) -> (13.3767, 21.9423)
  line L1532 (13.3767, 21.9423) -> (13.3496, 21.9901)
  line L1533 (13.3496, 21.9901) -> (13.3328, 22.0147)
  line L1534 (13.3328, 22.0147) -> (13.3136, 22.0395)
  line L1535 (13.3136, 22.0395) -> (13.2918, 22.0643)
  line L1536 (13.2918, 22.0643) -> (13.2674, 22.0888)
  line L1537 (13.2674, 22.0888) -> (13.24, 22.113)
  line L1538 (13.24, 22.113) -> (13.2096, 22.1366)
  line L1539 (13.2096, 22.1366) -> (13.176, 22.1595)
  line L1540 (13.176, 22.1595) -> (13.139, 22.1813)
  line L1541 (13.139, 22.1813) -> (13.0986, 22.202)
  line L1542 (13.0986, 22.202) -> (13.0544, 22.2214)
  line L1543 (13.0544, 22.2214) -> (13.0064, 22.2392)
  line L1544 (13.0064, 22.2392) -> (12.9544, 22.2552)
  line L1545 (12.9544, 22.2552) -> (12.8983, 22.2694)
  line L1546 (12.8983, 22.2694) -> (12.8378, 22.2813)
  line L1547 (12.8378, 22.2813) -> (12.7729, 22.291)
  line L1548 (12.7729, 22.291) -> (12.7033, 22.2981)
  line L1549 (12.7033, 22.2981) -> (12.629, 22.3026)
  line L1550 (12.629, 22.3026) -> (12.5496, 22.3041)
  line L1551 (12.5496, 22.3041) -> (9.3746, 22.3041)
  line L1552 (9.3746, 22.3041) -> (9.2869, 22.3056)
  line L1553 (9.2869, 22.3056) -> (9.2022, 22.3102)
  line L1554 (9.2022, 22.3102) -> (9.1205, 22.3179)
  line L1555 (9.1205, 22.3179) -> (9.0418, 22.3285)
  line L1556 (9.0418, 22.3285) -> (8.9661, 22.342)
  line L1557 (8.9661, 22.342) -> (8.8933, 22.3585)
  line L1558 (8.8933, 22.3585) -> (8.8233, 22.3778)
  line L1559 (8.8233, 22.3778) -> (8.7562, 22.4)
  line L1560 (8.7562, 22.4) -> (8.6918, 22.4249)
  line L1561 (8.6918, 22.4249) -> (8.6302, 22.4526)
  line L1562 (8.6302, 22.4526) -> (8.5713, 22.4831)
  line L1563 (8.5713, 22.4831) -> (8.5151, 22.5162)
  line L1564 (8.5151, 22.5162) -> (8.4616, 22.5519)
  line L1565 (8.4616, 22.5519) -> (8.4106, 22.5902)
  line L1566 (8.4106, 22.5902) -> (8.3622, 22.6311)
  line L1567 (8.3622, 22.6311) -> (8.3163, 22.6745)
  line L1568 (8.3163, 22.6745) -> (8.2923, 22.6994)
  line L1569 (8.2923, 22.6994) -> (8.2697, 22.7246)
  line L1570 (8.2697, 22.7246) -> (8.2486, 22.75)
  line L1571 (8.2486, 22.75) -> (8.229, 22.7755)
  line L1572 (8.229, 22.7755) -> (8.2106, 22.8011)
  line L1573 (8.2106, 22.8011) -> (8.1936, 22.8266)
  line L1574 (8.1936, 22.8266) -> (8.1779, 22.8521)
  line L1575 (8.1779, 22.8521) -> (8.1633, 22.8775)
  line L1576 (8.1633, 22.8775) -> (8.15, 22.9026)
  line L1577 (8.15, 22.9026) -> (8.1377, 22.9275)
  line L1578 (8.1377, 22.9275) -> (8.1265, 22.9521)
  line L1579 (8.1265, 22.9521) -> (8.1163, 22.9763)
  line L1580 (8.1163, 22.9763) -> (8.0988, 23.0233)
  line L1581 (8.0988, 23.0233) -> (8.0848, 23.0681)
  line L1582 (8.0848, 23.0681) -> (8.0739, 23.11)
  line L1583 (8.0739, 23.11) -> (8.0657, 23.1486)
  line L1584 (8.0657, 23.1486) -> (8.0598, 23.1835)
  line L1585 (8.0598, 23.1835) -> (8.0558, 23.214)
  line L1586 (8.0558, 23.214) -> (8.0535, 23.2397)
  line L1587 (8.0535, 23.2397) -> (8.0522, 23.2601)
  line L1588 (8.0522, 23.2601) -> (8.0517, 23.283)
  line L1589 (8.0517, 23.283) -> (8.0517, 23.3889)
  line L1590 (8.0517, 23.3889) -> (8.0522, 23.4118)
  line L1591 (8.0522, 23.4118) -> (8.0558, 23.4579)
  line L1592 (8.0558, 23.4579) -> (8.0598, 23.4884)
  line L1593 (8.0598, 23.4884) -> (8.0657, 23.5233)
  line L1594 (8.0657, 23.5233) -> (8.0739, 23.5619)
  line L1595 (8.0739, 23.5619) -> (8.0848, 23.6038)
  line L1596 (8.0848, 23.6038) -> (8.0988, 23.6486)
  line L1597 (8.0988, 23.6486) -> (8.1163, 23.6956)
  line L1598 (8.1163, 23.6956) -> (8.1377, 23.7444)
  line L1599 (8.1377, 23.7444) -> (8.1633, 23.7944)
  line L1600 (8.1633, 23.7944) -> (8.1936, 23.8453)
  line L1601 (8.1936, 23.8453) -> (8.229, 23.8964)
  line L1602 (8.229, 23.8964) -> (8.2486, 23.9219)
  line L1603 (8.2486, 23.9219) -> (8.2697, 23.9473)
  line L1604 (8.2697, 23.9473) -> (8.2923, 23.9725)
  line L1605 (8.2923, 23.9725) -> (8.3163, 23.9974)
  line L1606 (8.3163, 23.9974) -> (8.3622, 24.0408)
  line L1607 (8.3622, 24.0408) -> (8.4106, 24.0817)
  line L1608 (8.4106, 24.0817) -> (8.4616, 24.12)
  line L1609 (8.4616, 24.12) -> (8.5151, 24.1557)
  line L1610 (8.5151, 24.1557) -> (8.5713, 24.1888)
  line L1611 (8.5713, 24.1888) -> (8.6302, 24.2193)
  line L1612 (8.6302, 24.2193) -> (8.6918, 24.247)
  line L1613 (8.6918, 24.247) -> (8.7562, 24.2719)
  line L1614 (8.7562, 24.2719) -> (8.8233, 24.2941)
  line L1615 (8.8233, 24.2941) -> (8.8933, 24.3134)
  line L1616 (8.8933, 24.3134) -> (8.9661, 24.3299)
  line L1617 (8.9661, 24.3299) -> (9.0418, 24.3434)
  line L1618 (9.0418, 24.3434) -> (9.1205, 24.354)
  line L1619 (9.1205, 24.354) -> (9.2022, 24.3617)
  line L1620 (9.2022, 24.3617) -> (9.2869, 24.3663)
  line L1621 (9.2869, 24.3663) -> (9.3746, 24.3678)
  line L1622 (9.3746, 24.3678) -> (12.5232, 24.3678)
  line L1623 (12.5232, 24.3678) -> (12.6069, 24.3657)
  line L1624 (44.019, 23.5735) -> (44.055, 23.5717)
  line L1625 (44.055, 23.5717) -> (44.0904, 23.5687)
  line L1626 (44.0904, 23.5687) -> (44.125, 23.5646)
  line L1627 (44.125, 23.5646) -> (44.159, 23.5595)
  line L1628 (44.159, 23.5595) -> (44.1923, 23.5533)
  line L1629 (44.1923, 23.5533) -> (44.257, 23.5381)
  line L1630 (44.257, 23.5381) -> (44.3195, 23.5193)
  line L1631 (44.3195, 23.5193) -> (44.3798, 23.4973)
  line L1632 (44.3798, 23.4973) -> (44.4381, 23.4725)
  line L1633 (44.4381, 23.4725) -> (44.4948, 23.4451)
  line L1634 (44.4948, 23.4451) -> (44.5498, 23.4155)
  line L1635 (44.5498, 23.4155) -> (44.6035, 23.3842)
  line L1636 (44.6035, 23.3842) -> (44.6561, 23.3513)
  line L1637 (44.6561, 23.3513) -> (44.7077, 23.3173)
  line L1638 (44.7077, 23.3173) -> (44.8087, 23.2474)
  line L1639 (44.8087, 23.2474) -> (44.9082, 23.1772)
  line L1640 (44.9082, 23.1772) -> (45.0152, 23.0994)
  line L1641 (45.0152, 23.0994) -> (45.1198, 23.0259)
  line L1642 (45.1198, 23.0259) -> (45.172, 22.9914)
  line L1643 (45.172, 22.9914) -> (45.2244, 22.9586)
  line L1644 (45.2244, 22.9586) -> (45.2775, 22.9279)
  line L1645 (45.2775, 22.9279) -> (45.3315, 22.8994)
  line L1646 (45.3315, 22.8994) -> (45.3867, 22.8734)
  line L1647 (45.3867, 22.8734) -> (45.4435, 22.8501)
  line L1648 (45.4435, 22.8501) -> (45.5022, 22.8297)
  line L1649 (45.5022, 22.8297) -> (45.563, 22.8126)
  line L1650 (45.563, 22.8126) -> (45.6263, 22.7988)
  line L1651 (45.6263, 22.7988) -> (45.6924, 22.7887)
  line L1652 (45.6924, 22.7887) -> (45.7616, 22.7825)
  line L1653 (45.7616, 22.7825) -> (45.8342, 22.7803)
  line L1654 (45.8342, 22.7803) -> (46.3369, 22.7803)
  line L1655 (46.3369, 22.7803) -> (46.3369, 22.3305)
  line L1656 (46.3369, 22.3305) -> (45.8342, 22.3305)
  line L1657 (45.8342, 22.3305) -> (45.7851, 22.3314)
  line L1658 (45.7851, 22.3314) -> (45.7371, 22.3339)
  line L1659 (45.7371, 22.3339) -> (45.6902, 22.3379)
  line L1660 (45.6902, 22.3379) -> (45.6442, 22.3435)
  line L1661 (45.6442, 22.3435) -> (45.5992, 22.3504)
  line L1662 (45.5992, 22.3504) -> (45.5552, 22.3588)
  line L1663 (45.5552, 22.3588) -> (45.5121, 22.3684)
  line L1664 (45.5121, 22.3684) -> (45.47, 22.3793)
  line L1665 (45.47, 22.3793) -> (45.4287, 22.3914)
  line L1666 (45.4287, 22.3914) -> (45.3883, 22.4045)
  line L1667 (45.3883, 22.4045) -> (45.3101, 22.4338)
  line L1668 (45.3101, 22.4338) -> (45.2349, 22.4666)
  line L1669 (45.2349, 22.4666) -> (45.1628, 22.5025)
  line L1670 (45.1628, 22.5025) -> (45.0935, 22.5409)
  line L1671 (45.0935, 22.5409) -> (45.0268, 22.5812)
  line L1672 (45.0268, 22.5812) -> (44.9624, 22.6229)
  line L1673 (44.9624, 22.6229) -> (44.9003, 22.6654)
  line L1674 (44.9003, 22.6654) -> (44.7819, 22.7509)
  line L1675 (44.7819, 22.7509) -> (44.67, 22.8332)
  line L1676 (44.67, 22.8332) -> (44.583, 22.9001)
  line L1677 (44.583, 22.9001) -> (44.4997, 22.961)
  line L1678 (44.4997, 22.961) -> (44.4591, 22.9889)
  line L1679 (44.4591, 22.9889) -> (44.4189, 23.0151)
  line L1680 (44.4189, 23.0151) -> (44.379, 23.0393)
  line L1681 (44.379, 23.0393) -> (44.3393, 23.0614)
  line L1682 (44.3393, 23.0614) -> (44.2996, 23.0814)
  line L1683 (44.2996, 23.0814) -> (44.2597, 23.0991)
  line L1684 (44.2597, 23.0991) -> (44.2195, 23.1144)
  line L1685 (44.2195, 23.1144) -> (44.1789, 23.1272)
  line L1686 (44.1789, 23.1272) -> (44.1376, 23.1373)
  line L1687 (44.1376, 23.1373) -> (44.0956, 23.1447)
  line L1688 (44.0956, 23.1447) -> (44.0526, 23.1492)
  line L1689 (44.0526, 23.1492) -> (44.0086, 23.1507)
  line L1690 (44.0086, 23.1507) -> (43.9645, 23.1492)
  line L1691 (43.9645, 23.1492) -> (43.9216, 23.1447)
  line L1692 (43.9216, 23.1447) -> (43.8795, 23.1373)
  line L1693 (43.8795, 23.1373) -> (43.8383, 23.1272)
  line L1694 (43.8383, 23.1272) -> (43.7976, 23.1144)
  line L1695 (43.7976, 23.1144) -> (43.7574, 23.0991)
  line L1696 (43.7574, 23.0991) -> (43.7176, 23.0814)
  line L1697 (43.7176, 23.0814) -> (43.6779, 23.0614)
  line L1698 (43.6779, 23.0614) -> (43.6381, 23.0393)
  line L1699 (43.6381, 23.0393) -> (43.5983, 23.0151)
  line L1700 (43.5983, 23.0151) -> (43.5581, 22.9889)
  line L1701 (43.5581, 22.9889) -> (43.5174, 22.961)
  line L1702 (43.5174, 22.961) -> (43.4341, 22.9001)
  line L1703 (43.4341, 22.9001) -> (43.3471, 22.8332)
  line L1704 (43.3471, 22.8332) -> (43.2352, 22.7433)
  line L1705 (43.2352, 22.7433) -> (43.1169, 22.6542)
  line L1706 (43.1169, 22.6542) -> (43.0547, 22.6111)
  line L1707 (43.0547, 22.6111) -> (42.9904, 22.5695)
  line L1708 (42.9904, 22.5695) -> (42.9237, 22.5299)
  line L1709 (42.9237, 22.5299) -> (42.8543, 22.4926)
  line L1710 (42.8543, 22.4926) -> (42.7822, 22.4581)
  line L1711 (42.7822, 22.4581) -> (42.7071, 22.4268)
  line L1712 (42.7071, 22.4268) -> (42.6288, 22.3992)
  line L1713 (42.6288, 22.3992) -> (42.5472, 22.3756)
  line L1714 (42.5472, 22.3756) -> (42.462, 22.3565)
  line L1715 (42.462, 22.3565) -> (42.373, 22.3424)
  line L1716 (42.373, 22.3424) -> (42.28, 22.3336)
  line L1717 (42.28, 22.3336) -> (42.183, 22.3305)
  line L1718 (42.183, 22.3305) -> (41.6803, 22.3305)
  line L1719 (41.6803, 22.3305) -> (41.6803, 22.7803)
  line L1720 (41.6803, 22.7803) -> (42.183, 22.7803)
  line L1721 (42.183, 22.7803) -> (42.215, 22.7809)
  line L1722 (42.215, 22.7809) -> (42.2465, 22.7827)
  line L1723 (42.2465, 22.7827) -> (42.2777, 22.7857)
  line L1724 (42.2777, 22.7857) -> (42.3084, 22.7898)
  line L1725 (42.3084, 22.7898) -> (42.3387, 22.7949)
  line L1726 (42.3387, 22.7949) -> (42.3686, 22.8011)
  line L1727 (42.3686, 22.8011) -> (42.4273, 22.8163)
  line L1728 (42.4273, 22.8163) -> (42.4846, 22.8351)
  line L1729 (42.4846, 22.8351) -> (42.5406, 22.8571)
  line L1730 (42.5406, 22.8571) -> (42.5955, 22.8819)
  line L1731 (42.5955, 22.8819) -> (42.6493, 22.9093)
  line L1732 (42.6493, 22.9093) -> (42.7022, 22.9389)
  line L1733 (42.7022, 22.9389) -> (42.7542, 22.9702)
  line L1734 (42.7542, 22.9702) -> (42.8056, 23.0031)
  line L1735 (42.8056, 23.0031) -> (42.8564, 23.0371)
  line L1736 (42.8564, 23.0371) -> (43.0561, 23.1772)
  line L1737 (43.0561, 23.1772) -> (43.1556, 23.255)
  line L1738 (43.1556, 23.255) -> (43.2058, 23.2924)
  line L1739 (43.2058, 23.2924) -> (43.2566, 23.3285)
  line L1740 (43.2566, 23.3285) -> (43.3082, 23.363)
  line L1741 (43.3082, 23.363) -> (43.3607, 23.3958)
  line L1742 (43.3607, 23.3958) -> (43.4144, 23.4265)
  line L1743 (43.4144, 23.4265) -> (43.4695, 23.455)
  line L1744 (43.4695, 23.455) -> (43.5261, 23.481)
  line L1745 (43.5261, 23.481) -> (43.5845, 23.5043)
  line L1746 (43.5845, 23.5043) -> (43.6448, 23.5247)
  line L1747 (43.6448, 23.5247) -> (43.7072, 23.5418)
  line L1748 (43.7072, 23.5418) -> (43.772, 23.5556)
  line L1749 (43.772, 23.5556) -> (43.8392, 23.5657)
  line L1750 (43.8392, 23.5657) -> (43.9092, 23.5719)
  line L1751 (43.9092, 23.5719) -> (43.9821, 23.5741)
  line L1752 (43.9821, 23.5741) -> (44.019, 23.5735)
  line L1753 (38.9342, 38.6036) -> (38.9342, 32.2536)
  line L1754 (38.9342, 32.2536) -> (49.6022, 32.2536)
  line L1755 (49.6022, 38.6036) -> (38.9342, 38.6036)
  line L1756 (49.6022, 32.2536) -> (49.6022, 38.6036)
  line L1757 (25.9459, 45.6034) -> (25.9459, 39.2534)
  line L1758 (25.9459, 39.2534) -> (36.6139, 39.2534)
  line L1759 (36.6139, 45.6034) -> (25.9459, 45.6034)
  line L1760 (36.6139, 39.2534) -> (36.6139, 45.6034)
  line L1761 (38.9401, 50.4289) -> (38.9401, 44.3329)
  line L1762 (38.9401, 44.3329) -> (46.8141, 44.3329)
  line L1763 (46.8141, 50.4289) -> (38.9401, 50.4289)
  line L1764 (46.8141, 44.3329) -> (46.8141, 50.4289)
  line L1765 (19.1669, 17.9808) -> (19.1669, 9.0908)
  line L1766 (19.1669, 9.0908) -> (42.0268, 9.0908)
  line L1767 (42.0268, 17.9808) -> (19.1669, 17.9808)
  line L1768 (42.0268, 9.0908) -> (42.0268, 17.9808)
  line L1769 (27.3429, 54.8247) -> (27.3429, 48.7287)
  line L1770 (27.3429, 48.7287) -> (35.2169, 48.7287)
  line L1771 (35.2169, 54.8247) -> (27.3429, 54.8247)
  line L1772 (35.2169, 48.7287) -> (35.2169, 54.8247)
  line L1773 (27.3429, 33.5236) -> (27.3429, 27.4276)
  line L1774 (27.3429, 27.4276) -> (35.2169, 27.4276)
  line L1775 (35.2169, 33.5236) -> (27.3429, 33.5236)
  line L1776 (35.2169, 27.4276) -> (35.2169, 33.5236)
  line L1777 (10.9942, 38.6036) -> (10.9942, 32.2536)
  line L1778 (10.9942, 32.2536) -> (21.6622, 32.2536)
  line L1779 (21.6622, 38.6036) -> (10.9942, 38.6036)
  line L1780 (21.6622, 32.2536) -> (21.6622, 38.6036)
  line L1781 (13.7719, 50.3509) -> (13.7719, 44.2549)
  line L1782 (13.7719, 44.2549) -> (21.6459, 44.2549)
  line L1783 (21.6459, 50.3509) -> (13.7719, 50.3509)
  line L1784 (21.6459, 44.2549) -> (21.6459, 50.3509)
  line L1785 (0.175, 30.5116) -> (15.175, 4.5309)
  line L1786 (45.175, 4.5309) -> (60.175, 30.5116)
  line L1787 (15.175, 4.5309) -> (45.175, 4.5309)
  circle A36 centre (4.8982, 30.5264) radius 1.5
  circle A37 centre (17.5982, 53.3864) radius 1.5
  circle A38 centre (42.9982, 53.3864) radius 1.5
  line L1788 (60.175, 30.5116) -> (45.175, 56.4924)
  line L1789 (45.175, 56.4924) -> (15.175, 56.4924)
  line L1790 (15.175, 56.4924) -> (0.175, 30.5116)
  line L1791 (12.0832, 28.5364) -> (15.6832, 28.5364)
  line L1792 (15.6832, 28.5364) -> (15.6832, 27.4364)
  line L1793 (15.6832, 27.4364) -> (12.0832, 27.4364)
  line L1794 (12.0832, 27.4364) -> (12.0832, 28.5364)
  line L1795 (17.1632, 28.5364) -> (20.7632, 28.5364)
  line L1796 (20.7632, 28.5364) -> (20.7632, 27.4364)
  line L1797 (20.7632, 27.4364) -> (17.1632, 27.4364)
  line L1798 (17.1632, 27.4364) -> (17.1632, 28.5364)
  line L1799 (12.0832, 27.9864) -> (15.6832, 27.9864) construction
  line L1800 (26.6943, 36.1834) -> (30.2943, 36.1834)
  line L1801 (30.2943, 36.1834) -> (30.2943, 35.0834)
  line L1802 (30.2943, 35.0834) -> (26.6943, 35.0834)
  line L1803 (26.6943, 35.0834) -> (26.6943, 36.1834)
  line L1804 (31.7743, 36.1834) -> (35.3743, 36.1834)
  line L1805 (35.3743, 36.1834) -> (35.3743, 35.0834)
  line L1806 (35.3743, 35.0834) -> (31.7743, 35.0834)
  line L1807 (31.7743, 35.0834) -> (31.7743, 36.1834)
  line L1808 (40.0232, 28.5364) -> (43.6232, 28.5364)
  line L1809 (43.6232, 28.5364) -> (43.6232, 27.4364)
  line L1810 (43.6232, 27.4364) -> (40.0232, 27.4364)
  line L1811 (40.0232, 27.4364) -> (40.0232, 28.5364)
  line L1812 (45.1032, 28.5364) -> (48.7032, 28.5364)
  line L1813 (48.7032, 28.5364) -> (48.7032, 27.4364)
  line L1814 (48.7032, 27.4364) -> (45.1032, 27.4364)
  line L1815 (45.1032, 27.4364) -> (45.1032, 28.5364)
  line L1816 (30.175, 56.4924) -> (30.175, 4.5309) construction
  line L1817 (25.1331, 54.8247) -> (35.2169, 54.8247)
  line L1818 (35.2169, 54.8247) -> (35.2169, 48.7287)
  line L1819 (35.2169, 48.7287) -> (25.1331, 48.7287)
  line L1820 (25.1331, 48.7287) -> (25.1331, 54.8247)
  line L1821 (36.6139, 45.6034) -> (23.7361, 45.6034)